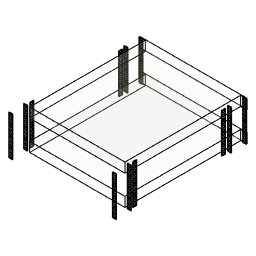
battery case (Autodesk Fusion 360 archive; units mm, degrees)
design "rack 19"
Autodesk Fusion 360 part; units mm, degrees
sketch "Sketch1" plane through (0, 0, 0) normal (0, 1, 0) x (1, 0, 0)
  line L0 (0, 0) -> (16.7, 0)
  line L1 (16.7, 0) -> (16.7, -177.8)
  line L2 (16.7, -177.8) -> (0, -177.8)
  line L3 (0, -177.8) -> (0, 0)
  line L4 (16.7, 0) -> (466.7, 0)
  line L5 (466.7, 0) -> (483.4, 0)
  line L6 (483.4, 0) -> (483.4, -177.8)
  line L7 (483.4, -177.8) -> (466.7, -177.8)
  line L8 (466.7, -177.8) -> (466.7, 0)
  line L9 (0, -88.9) -> (16.7, -88.9)
  line L10 (0, -88.9) -> (0, 0)
  line L11 (0, -44.45) -> (16.7, -44.45)
  line L12 (0, -88.9) -> (0, -177.8)
  line L13 (0, -133.35) -> (16.7, -133.35)
  line L14 (0, -88.9) -> (0, -44.45)
  line L15 (0, -66.675) -> (16.7, -66.675)
  line L16 (8.35, -66.675) -> (8.35, -82.55)
  line L17 (8.35, -66.675) -> (8.35, -50.8)
  line L18 (3.85, -87.05) -> (12.85, -87.05)
  line L19 (12.85, -87.05) -> (12.85, -78.05)
  line L20 (12.85, -78.05) -> (3.85, -78.05)
  line L21 (3.85, -78.05) -> (3.85, -87.05)
  line L22 (3.85, -87.05) -> (12.85, -78.05) construction
  line L23 (12.85, -87.05) -> (3.85, -78.05) construction
  line L24 (3.85, -71.175) -> (12.85, -71.175)
  line L25 (12.85, -71.175) -> (12.85, -62.175)
  line L26 (12.85, -62.175) -> (3.85, -62.175)
  line L27 (3.85, -62.175) -> (3.85, -71.175)
  line L28 (3.85, -71.175) -> (12.85, -62.175) construction
  line L29 (12.85, -71.175) -> (3.85, -62.175) construction
  line L30 (3.85, -55.3) -> (12.85, -55.3)
  line L31 (12.85, -55.3) -> (12.85, -46.3)
  line L32 (12.85, -46.3) -> (3.85, -46.3)
  line L33 (3.85, -46.3) -> (3.85, -55.3)
  line L34 (3.85, -55.3) -> (12.85, -46.3) construction
  line L35 (12.85, -55.3) -> (3.85, -46.3) construction
  line L36 (3.85, -10.85) -> (3.85, -1.85)
  line L37 (12.85, -42.6) -> (3.85, -42.6)
  line L38 (3.85, -17.725) -> (12.85, -26.725) construction
  line L39 (3.85, -33.6) -> (12.85, -33.6)
  line L40 (3.85, -1.85) -> (12.85, -10.85) construction
  line L41 (12.85, -1.85) -> (3.85, -10.85) construction
  line L42 (3.85, -33.6) -> (12.85, -42.6) construction
  line L43 (3.85, -1.85) -> (12.85, -1.85)
  line L44 (12.85, -10.85) -> (3.85, -10.85)
  line L45 (12.85, -17.725) -> (12.85, -26.725)
  line L46 (3.85, -17.725) -> (12.85, -17.725)
  line L47 (3.85, -26.725) -> (3.85, -17.725)
  line L48 (8.35, -22.225) -> (8.35, -38.1)
  line L49 (12.85, -17.725) -> (3.85, -26.725) construction
  line L50 (12.85, -33.6) -> (3.85, -42.6) construction
  line L51 (12.85, -1.85) -> (12.85, -10.85)
  line L52 (12.85, -33.6) -> (12.85, -42.6)
  line L53 (8.35, -22.225) -> (8.35, -6.35)
  line L54 (3.85, -42.6) -> (3.85, -33.6)
  line L55 (12.85, -26.725) -> (3.85, -26.725)
  line L56 (3.85, -166.95) -> (3.85, -175.95)
  line L57 (3.85, -90.75) -> (12.85, -99.75) construction
  line L58 (12.85, -99.75) -> (3.85, -99.75)
  line L59 (3.85, -131.5) -> (3.85, -122.5)
  line L60 (12.85, -166.95) -> (3.85, -166.95)
  line L61 (3.85, -90.75) -> (12.85, -90.75)
  line L62 (3.85, -99.75) -> (3.85, -90.75)
  line L63 (12.85, -106.625) -> (12.85, -115.625)
  line L64 (3.85, -160.075) -> (12.85, -160.075)
  line L65 (3.85, -135.2) -> (3.85, -144.2)
  line L66 (12.85, -175.95) -> (12.85, -166.95)
  line L67 (8.35, -111.125) -> (8.35, -127)
  line L68 (12.85, -122.5) -> (12.85, -131.5)
  line L69 (3.85, -106.625) -> (12.85, -106.625)
  line L70 (12.85, -106.625) -> (3.85, -115.625) construction
  line L71 (12.85, -160.075) -> (3.85, -151.075) construction
  line L72 (12.85, -90.75) -> (12.85, -99.75)
  line L73 (12.85, -90.75) -> (3.85, -99.75) construction
  line L74 (3.85, -175.95) -> (12.85, -166.95) construction
  line L75 (12.85, -175.95) -> (3.85, -166.95) construction
  line L76 (12.85, -122.5) -> (3.85, -131.5) construction
  line L77 (12.85, -115.625) -> (3.85, -115.625)
  line L78 (3.85, -144.2) -> (12.85, -144.2)
  line L79 (3.85, -122.5) -> (12.85, -131.5) construction
  line L80 (12.85, -135.2) -> (3.85, -135.2)
  line L81 (8.35, -155.575) -> (8.35, -139.7)
  line L82 (3.85, -122.5) -> (12.85, -122.5)
  line L83 (12.85, -131.5) -> (3.85, -131.5)
  line L84 (3.85, -115.625) -> (3.85, -106.625)
  line L85 (3.85, -175.95) -> (12.85, -175.95)
  line L86 (8.35, -155.575) -> (8.35, -171.45)
  line L87 (12.85, -160.075) -> (12.85, -151.075)
  line L88 (8.35, -111.125) -> (8.35, -95.25)
  line L89 (3.85, -160.075) -> (12.85, -151.075) construction
  line L90 (3.85, -144.2) -> (12.85, -135.2) construction
  line L91 (12.85, -144.2) -> (3.85, -135.2) construction
  line L92 (12.85, -151.075) -> (3.85, -151.075)
  line L93 (3.85, -106.625) -> (12.85, -115.625) construction
  line L94 (12.85, -144.2) -> (12.85, -135.2)
  line L95 (3.85, -151.075) -> (3.85, -160.075)
  line L96 (241.7, 0) -> (241.7, -10)
  line L97 (470.55, -122.5) -> (479.55, -131.5) construction
  line L98 (470.55, -78.05) -> (479.55, -78.05)
  line L99 (470.55, -106.625) -> (479.55, -115.625) construction
  line L100 (475.05, -111.125) -> (475.05, -127)
  line L101 (479.55, -122.5) -> (470.55, -131.5) construction
  line L102 (479.55, -122.5) -> (470.55, -122.5)
  line L103 (470.55, -106.625) -> (470.55, -115.625)
  line L104 (470.55, -166.95) -> (479.55, -166.95)
  line L105 (479.55, -87.05) -> (470.55, -87.05)
  line L106 (479.55, -115.625) -> (479.55, -106.625)
  line L107 (479.55, -87.05) -> (470.55, -78.05) construction
  line L108 (475.05, -22.225) -> (475.05, -6.35)
  line L109 (470.55, -62.175) -> (479.55, -62.175)
  line L110 (470.55, -115.625) -> (479.55, -115.625)
  line L111 (475.05, -111.125) -> (475.05, -95.25)
  line L112 (470.55, -55.3) -> (479.55, -46.3) construction
  line L113 (470.55, -71.175) -> (479.55, -62.175) construction
  line L114 (479.55, -10.85) -> (479.55, -1.85)
  line L115 (479.55, -166.95) -> (479.55, -175.95)
  line L116 (470.55, -55.3) -> (470.55, -46.3)
  line L117 (470.55, -175.95) -> (479.55, -166.95) construction
  line L118 (479.55, -1.85) -> (470.55, -1.85)
  line L119 (479.55, -26.725) -> (479.55, -17.725)
  line L120 (470.55, -42.6) -> (479.55, -42.6)
  line L121 (479.55, -55.3) -> (470.55, -46.3) construction
  line L122 (470.55, -175.95) -> (470.55, -166.95)
  line L123 (470.55, -131.5) -> (479.55, -131.5)
  line L124 (470.55, -144.2) -> (470.55, -135.2)
  line L125 (475.05, -66.675) -> (475.05, -50.8)
  line L126 (479.55, -62.175) -> (479.55, -71.175)
  line L127 (470.55, -160.075) -> (479.55, -151.075) construction
  line L128 (479.55, -71.175) -> (470.55, -71.175)
  line L129 (475.05, -155.575) -> (475.05, -139.7)
  line L130 (479.55, -151.075) -> (479.55, -160.075)
  line L131 (479.55, -175.95) -> (470.55, -175.95)
  line L132 (470.55, -135.2) -> (479.55, -135.2)
  line L133 (479.55, -1.85) -> (470.55, -10.85) construction
  line L134 (470.55, -17.725) -> (479.55, -26.725) construction
  line L135 (470.55, -90.75) -> (479.55, -99.75) construction
  line L136 (479.55, -135.2) -> (479.55, -144.2)
  line L137 (479.55, -106.625) -> (470.55, -106.625)
  line L138 (475.05, -22.225) -> (475.05, -38.1)
  line L139 (479.55, -90.75) -> (470.55, -90.75)
  line L140 (470.55, -10.85) -> (479.55, -10.85)
  line L141 (479.55, -42.6) -> (479.55, -33.6)
  line L142 (479.55, -33.6) -> (470.55, -42.6) construction
  line L143 (470.55, -1.85) -> (470.55, -10.85)
  line L144 (479.55, -160.075) -> (470.55, -160.075)
  line L145 (479.55, -90.75) -> (470.55, -99.75) construction
  line L146 (479.55, -99.75) -> (479.55, -90.75)
  line L147 (479.55, -55.3) -> (470.55, -55.3)
  line L148 (470.55, -122.5) -> (470.55, -131.5)
  line L149 (470.55, -26.725) -> (479.55, -26.725)
  line L150 (470.55, -160.075) -> (470.55, -151.075)
  line L151 (479.55, -144.2) -> (470.55, -144.2)
  line L152 (470.55, -71.175) -> (470.55, -62.175)
  line L153 (479.55, -78.05) -> (479.55, -87.05)
  line L154 (470.55, -87.05) -> (470.55, -78.05)
  line L155 (479.55, -46.3) -> (479.55, -55.3)
  line L156 (479.55, -144.2) -> (470.55, -135.2) construction
  line L157 (479.55, -131.5) -> (479.55, -122.5)
  line L158 (479.55, -71.175) -> (470.55, -62.175) construction
  line L159 (470.55, -151.075) -> (479.55, -151.075)
  line L160 (470.55, -144.2) -> (479.55, -135.2) construction
  line L161 (479.55, -160.075) -> (470.55, -151.075) construction
  line L162 (475.05, -155.575) -> (475.05, -171.45)
  line L163 (479.55, -175.95) -> (470.55, -166.95) construction
  line L164 (470.55, -17.725) -> (470.55, -26.725)
  line L165 (470.55, -87.05) -> (479.55, -78.05) construction
  line L166 (479.55, -106.625) -> (470.55, -115.625) construction
  line L167 (470.55, -99.75) -> (479.55, -99.75)
  line L168 (475.05, -66.675) -> (475.05, -82.55)
  line L169 (470.55, -90.75) -> (470.55, -99.75)
  line L170 (479.55, -33.6) -> (470.55, -33.6)
  line L171 (470.55, -1.85) -> (479.55, -10.85) construction
  line L172 (470.55, -33.6) -> (479.55, -42.6) construction
  line L173 (479.55, -17.725) -> (470.55, -26.725) construction
  line L174 (470.55, -33.6) -> (470.55, -42.6)
  line L175 (479.55, -17.725) -> (470.55, -17.725)
  line L176 (470.55, -46.3) -> (479.55, -46.3)
  point P0 (8.35, -82.55)
  point P1 (8.35, -66.675)
  point P2 (8.35, -50.8)
  point P3 (8.35, -22.225)
  point P4 (8.35, -6.35)
  point P5 (8.35, -38.1)
  point P6 (8.35, -171.45)
  point P7 (8.35, -95.25)
  point P8 (8.35, -111.125)
  point P9 (8.35, -139.7)
  point P10 (8.35, -155.575)
  point P11 (8.35, -127)
  point P12 (475.05, -95.25)
  point P13 (475.05, -111.125)
  point P14 (475.05, -155.575)
  point P15 (475.05, -66.675)
  point P16 (475.05, -127)
  point P17 (475.05, -6.35)
  point P18 (475.05, -82.55)
  point P19 (475.05, -22.225)
  point P20 (475.05, -50.8)
  point P21 (475.05, -139.7)
  point P22 (475.05, -38.1)
  point P23 (475.05, -171.45)
  dimension "d1" = 16.7
  dimension "d2" = 177.8
  dimension "d3" = 450
  dimension "d4" = 16.7
  dimension "d5" = 177.8
  dimension "d6" = 15.875
  dimension "d7" = 15.875
  dimension "d8" = 9
  dimension "d9" = 9
  dimension "d10" = 9
  dimension "d11" = 9
  dimension "d12" = 9
  dimension "d13" = 9
  constraint horizontal L0
  constraint vertical L1
  constraint horizontal L2
  constraint vertical L3
  constraint coincident L0.start L3.end
  constraint perpendicular L1 L4
  constraint horizontal L5
  constraint vertical L6
  constraint horizontal L7
  constraint vertical L8
  constraint midpoint L3 L9.start
  constraint midpoint L1 L9.end
  constraint midpoint L10 L11.start
  constraint coincident L1 L11.end
  constraint perpendicular L1 L11
  constraint midpoint L12 L13.start
  constraint coincident L1 L13.end
  constraint perpendicular L1 L13
  constraint midpoint L14 L15.start
  constraint coincident L1 L15.end
  constraint perpendicular L1 L15
  constraint midpoint L15 P1
  constraint perpendicular L15 L16
  constraint parallel L14 L17
  constraint horizontal L18
  constraint perpendicular L18 L19
  constraint parallel L18 L20
  constraint parallel L19 L21
  constraint coincident L22 P0
  constraint coincident L23 P0
  constraint coincident P0 L16.end
  constraint horizontal L24
  constraint perpendicular L24 L25
  constraint parallel L24 L26
  constraint parallel L25 L27
  constraint coincident L28 P1
  constraint coincident L29 P1
  constraint coincident P1 L16.start
  constraint horizontal L30
  constraint perpendicular L30 L31
  constraint parallel L30 L32
  constraint parallel L31 L33
  constraint coincident L34 P2
  constraint coincident L35 P2
  constraint coincident P2 L17.end
  constraint symmetric L11 P1 P3
  constraint symmetric L11 P0 P4
  constraint symmetric L11 P2 P5
  constraint symmetric L11 L18.start L36.end
  constraint symmetric L11 L18.end L41.start
  constraint symmetric L11 L19.end L40.end
  constraint symmetric L11 L20.end L36.start
  constraint symmetric L11 L24.start L38.start
  constraint symmetric L11 L24.end L45.start
  constraint symmetric L11 L25.end L38.end
  constraint symmetric L11 L26.end L47.start
  constraint symmetric L11 L30.start L39.start
  constraint symmetric L11 L30.end L39.end
  constraint symmetric L11 L31.end L37.start
  constraint symmetric L11 L32.end L37.end
  constraint symmetric L9 P1 P8
  constraint symmetric L9 P0 P7
  constraint symmetric L9 P2 P11
  constraint symmetric L9 L18.start L57.start
  constraint symmetric L9 L18.end L61.end
  constraint symmetric L9 L19.end L57.end
  constraint symmetric L9 L20.end L58.end
  constraint symmetric L9 L24.start L69.start
  constraint symmetric L9 L24.end L63.start
  constraint symmetric L9 L25.end L63.end
  constraint symmetric L9 L26.end L70.end
  constraint symmetric L9 L30.start L59.end
  constraint symmetric L9 L30.end L68.start
  constraint symmetric L9 L31.end L68.end
  constraint symmetric L9 L32.end L59.start
  constraint symmetric L9 L40.end L60.start
  constraint symmetric L9 L41.start L66.start
  constraint symmetric L9 L36.start L56.start
  constraint symmetric L9 L36.end L56.end
  constraint symmetric L9 P5 P9
  constraint symmetric L9 P3 P10
  constraint symmetric L9 L39.start L65.end
  constraint symmetric L9 P4 P6
  constraint symmetric L9 L45.start L64.end
  constraint symmetric L9 L38.start L64.start
  constraint symmetric L9 L38.end L87.end
  constraint symmetric L9 L47.start L71.end
  constraint symmetric L9 L37.end L65.start
  constraint symmetric L9 L37.start L80.start
  constraint symmetric L9 L39.end L78.end
  constraint midpoint L4 L96.start
  constraint perpendicular L4 L96
  constraint symmetric P1 L96 P15
  constraint symmetric P0 L96 P18
  constraint symmetric P2 L96 L125.end
  constraint symmetric L18.start L96 L105.start
  constraint symmetric L18.end L96 L105.end
  constraint symmetric L19.end L96 L98.start
  constraint symmetric L20.end L96 L98.end
  constraint symmetric L24.start L96 L126.end
  constraint symmetric L24.end L96 L113.start
  constraint symmetric L25.end L96 L109.start
  constraint symmetric L26.end L96 L109.end
  constraint symmetric L30.start L96 L121.start
  constraint symmetric L30.end L96 L112.start
  constraint symmetric L31.end L96 L116.end
  constraint symmetric L32.end L96 L112.end
  constraint symmetric P2 L96 P20
  constraint symmetric L40.end L96 L133.end
  constraint symmetric L41.start L96 L118.end
  constraint symmetric L36.start L96 L114.start
  constraint symmetric L36.end L96 L114.end
  constraint symmetric P5 L96 P22
  constraint symmetric P3 L96 P19
  constraint symmetric L39.start L96 L141.end
  constraint symmetric P4 L96 P17
  constraint symmetric L45.start L96 L134.start
  constraint symmetric L38.start L96 L119.end
  constraint symmetric L38.end L96 L149.start
  constraint symmetric L47.start L96 L119.start
  constraint symmetric L37.end L96 L120.end
  constraint symmetric L37.start L96 L120.start
  constraint symmetric L39.end L96 L170.end
  constraint symmetric L66.start L96 L117.start
  constraint symmetric L59.start L96 L97.end
  constraint symmetric L63.end L96 L103.end
  constraint symmetric L60.start L96 L104.start
  constraint symmetric L68.end L96 L101.end
  constraint symmetric L63.start L96 L99.start
  constraint symmetric P11 L96 P16
  constraint symmetric L56.end L96 L115.end
  constraint symmetric L65.end L96 L136.end
  constraint symmetric P10 L96 P14
  constraint symmetric L56.start L96 L104.end
  constraint symmetric L69.start L96 L106.end
  constraint symmetric P7 L96 P12
  constraint symmetric P9 L96 P21
  constraint symmetric P6 L96 P23
  constraint symmetric L64.start L96 L130.end
  constraint symmetric P8 L96 P13
  constraint symmetric L71.end L96 L127.end
  constraint symmetric L64.end L96 L127.start
  constraint symmetric L57.start L96 L139.start
  constraint symmetric L87.end L96 L150.end
  constraint symmetric L59.end L96 L101.start
  constraint symmetric L68.start L96 L97.start
  constraint symmetric L70.end L96 L99.end
  constraint symmetric L65.start L96 L132.end
  constraint symmetric L61.end L96 L135.start
  constraint symmetric L80.start L96 L124.end
  constraint symmetric L57.end L96 L145.end
  constraint symmetric L78.end L96 L124.start
  constraint symmetric L58.end L96 L135.end
  measures "d1" distance of L0.start L0.end
  measures "d2" distance of L0.start L2.end
  measures "d3" distance of L0.end L4.end
  measures "d4" distance of L4.end L5.end
  measures "d5" distance of L4.end L7.end
  measures "d6" distance of P1 P0
  measures "d7" distance of P1 P2
  measures "d8" distance of L19.end L20.end
  measures "d9" distance of L18.end L19.end
  measures "d10" distance of L25.end L26.end
  measures "d11" distance of L24.end L25.end
  measures "d12" distance of L31.end L32.end
  measures "d13" distance of L30.end L31.end
extrude "Extrude1" add sketch "Sketch1" against normal blind 2 contours L0 L1 L3 L10 L11 | L1 L3 L10 L11 L14 L15 L25 L26 L27 | L1 L3 L9 L10 L14 L15 L24 L25 L27 | L1 L3 L9 L12 L13 | L1 L2 L3 L12 L13 | L5 L6 L7 L8 makes body 1 at (9.85, 0, 59.8833) makes body 2 at (476.55, 0, 31.3083)
sketch "Sketch2" plane through (0, 0, 0) normal (0, 1, 0) x (1, 0, 0)
  line L0 (241.7, -0.5) -> (241.7, -10.5)
  line L1 (241.7, -0.5) -> (482.6, -0.5)
  line L2 (241.7, -0.5) -> (0.8, -0.5)
  line L3 (0.8, -0.5) -> (0.8, -44)
  line L4 (0.8, -44) -> (482.6, -44)
  line L5 (482.6, -44) -> (482.6, -0.5)
  line L6 (241.7, -44.95) -> (0.8, -44.95)
  line L7 (0.8, -44.95) -> (0.8, -88.45)
  line L8 (241.7, -44.95) -> (482.6, -44.95)
  line L9 (0.8, -88.45) -> (482.6, -88.45)
  line L10 (241.7, -44.95) -> (241.7, -54.95)
  line L11 (482.6, -88.45) -> (482.6, -44.95)
  line L12 (241.7, -133.85) -> (0.8, -133.85)
  line L13 (0.8, -133.85) -> (0.8, -177.35)
  line L14 (241.7, -133.85) -> (482.6, -133.85)
  line L15 (0.8, -177.35) -> (482.6, -177.35)
  line L16 (241.7, -133.85) -> (241.7, -143.85)
  line L17 (482.6, -177.35) -> (482.6, -133.85)
  line L18 (241.7, -0.5) -> (27.2, -0.5)
  line L19 (241.7, -0.5) -> (456.2, -0.5)
  line L20 (456.2, -0.5) -> (456.2, -44)
  line L21 (27.2, -0.5) -> (27.2, -44)
  line L22 (27.2, -44) -> (27.2, -177.35)
  line L23 (456.2, -44) -> (456.2, -177.35)
  point P0 (0, -44.45)
  point P1 (0, -133.35)
  dimension "d16" = 240.9
  dimension "d17" = 240.9
  dimension "d18" = 43.5
  dimension "d19" = 240.9
  dimension "d20" = 240.9
  dimension "d21" = 43.5
  dimension "d22" = 240.9
  dimension "d23" = 240.9
  dimension "d24" = 43.5
  dimension "d25" = 214.5
  dimension "d26" = 214.5
  constraint perpendicular L0 L1
  constraint perpendicular L0 L2
  constraint perpendicular L2 L3
  constraint perpendicular L3 L4
  constraint perpendicular L1 L5
  constraint perpendicular L8 L10
  constraint perpendicular L6 L10
  constraint perpendicular L6 L7
  constraint perpendicular L7 L9
  constraint perpendicular L8 L11
  constraint perpendicular L14 L16
  constraint perpendicular L12 L16
  constraint perpendicular L12 L13
  constraint perpendicular L13 L15
  constraint perpendicular L14 L17
  constraint perpendicular L0 L18
  constraint perpendicular L0 L19
  constraint coincident L4 L20.end
  constraint perpendicular L4 L20
  constraint coincident L4 L21.end
  constraint perpendicular L6 L21
  constraint coincident L15 L22.end
  constraint perpendicular L15 L22
  constraint coincident L15 L23.end
  constraint perpendicular L15 L23
  measures "d16" distance of L0.start L1.end
  measures "d17" distance of L0.start L2.end
  measures "d18" distance of L2.end L3.end
  measures "d19" distance of L6.start L8.end
  measures "d20" distance of L6.start L6.end
  measures "d21" distance of L7.end L6.end
  measures "d22" distance of L12.start L14.end
  measures "d23" distance of L12.start L12.end
  measures "d24" distance of L13.end L12.end
  measures "d25" distance of L0.start L18.end
  measures "d26" distance of L0.start L19.end
extrude "Extrude2" add sketch "Sketch2" along normal blind 2.5 separate body contours L1 L2 L4 L18 L19 L20 L21 | L1 L4 L5 L20 | L2 L3 L4 L21 | L6 L8 L9 L22 L23 | L8 L9 L11 L23 | L6 L7 L9 L22 | L12 L14 L15 L22 L23 | L14 L15 L17 L23 | L12 L13 L15 L22 makes body 3 at (161.4, 0, 15) makes body 4 at (161.4, 0, 59.45) makes body 5 at (161.4, 0, 148.35)
extrude "Extrude3" add sketch "Sketch2" against normal blind 230 contours L1 L2 L4 L18 L19 L20 L21 | L6 L8 L9 L22 L23 | L12 L14 L15 L22 L23 bodies 3 4 5
copy_body "CopyPasteBodies2" bodies 1 2 makes body 6 makes body 7
move_body "Move2" bodies 6 7 to x (1, 0, 0) y (0, 1, 0) z (0, 0, 1) at (0, -68, 0)
copy_body "CopyPasteBodies3" bodies 2 1 makes body 8 makes body 9
move_body "Move3" bodies 8 9 to x (1, 0, 0) y (0, 1, 0) z (0, 0, 1) at (0, -519, 0)
copy_body "CopyPasteBodies4" bodies 1 2 makes body 10 makes body 11
move_body "Move4" bodies 10 11 to x (1, 0, 0) y (0, 1, 0) z (0, 0, 1) at (0, -586, 0)
extrude "Extrude4" add 2 faces at (170.2, -230, 148.35) (170.2, -230, 29.5) along direction (0, -1, 0) blind 291 on bodies 3 5 bodies 5 3
sketch "Sketch3" plane through (0, 0, 0) normal (0, 0, 1) x (1, 0, 0)
  line L0 (466.7, -70) -> (466.7, -519)
  line L1 (466.7, -294.5) -> (466.7, -486)
  line L2 (466.7, -294.5) -> (466.7, -103)
  line L3 (16.7, -70) -> (16.7, -519)
  line L4 (466.7, -486) -> (16.7, -486)
  line L5 (466.7, -103) -> (16.7, -103)
  line L6 (12.85, -99.75) -> (3.85, -99.75)
  line L7 (8.35, -99.75) -> (16.15, -99.75)
  line L8 (16.15, -99.75) -> (11.15, -99.75)
  line L9 (11.15, -99.75) -> (11.15, -98.75)
  line L10 (16.7, -103) -> (11.15, -103)
  line L11 (16.7, -486) -> (11.15, -486)
  line L12 (466.7, -486) -> (472.25, -486)
  line L13 (466.7, -103) -> (472.25, -103)
  dimension "d33" = 191.5
  dimension "d34" = 191.5
  dimension "d35" = 7.8
  dimension "d36" = 5
  dimension "d37" = 1
  dimension "d38" = 5.55
  dimension "d39" = 5.55
  dimension "d40" = 5.55
  constraint vertical L0
  constraint midpoint L0 L1.start
  constraint parallel L0 L1
  constraint parallel L0 L2
  constraint parallel L0 L3
  constraint coincident L3 L4.end
  constraint perpendicular L3 L4
  constraint coincident L3 L5.end
  constraint perpendicular L3 L5
  constraint horizontal L6
  constraint midpoint L6 L7.start
  constraint parallel L6 L7
  constraint coincident L6 L8.end
  constraint perpendicular L7 L9
  constraint parallel L8 L10
  constraint perpendicular L3 L11
  constraint perpendicular L0 L12
  constraint perpendicular L0 L13
  measures "d33" distance of L1.start L1.end
  measures "d34" distance of L1.start L2.end
  measures "d35" distance of L7.start L7.end
  measures "d36" distance of L7.end L8.end
  measures "d37" distance of L8.end L9.end
  measures "d38" distance of L4.end L11.end
  measures "d39" distance of L1.end L12.end
  measures "d40" distance of L2.end L13.end
copy_body "CopyPasteBodies5" bodies 6 makes body 12
copy_body "CopyPasteBodies6" bodies 6 makes body 13
move_body "Move5" bodies 13 to x (0, 1, 0) y (-1, 0, 0) z (0, 0, 1) at (-58.85, -103, 0)
copy_body "CopyPasteBodies7" bodies 7 makes body 14
move_body "Move6" bodies 14 to x (0, 1, 0) y (-1, 0, 0) z (0, 0, 1) at (404.25, -569.7, 0)
copy_body "CopyPasteBodies8" bodies 13 14 makes body 15 makes body 16
move_body "Move7" bodies 15 16 to x (1, 0, 0) y (0, 1, 0) z (0, 0, 1) at (0, -399.7, 0)
hidden bodies 4
equation "d16 = ( 481.8 / 2 ) * 1 mm"
equation "d17 = ( 481.8 / 2 ) * 1 mm"
equation "d19 = ( 481.8 / 2 ) * 1 mm"
equation "d20 = ( 481.8 / 2 ) * 1 mm"
equation "d22 = ( 481.8 / 2 ) * 1 mm"
equation "d23 = ( 481.8 / 2 ) * 1 mm"
equation "d25 = ( 429 / 2 ) * 1 mm"
equation "d26 = ( 429 / 2 ) * 1 mm"
equation "d33 = ( 383 / 2 ) * 1 mm"
equation "d34 = ( 383 / 2 ) * 1 mm"

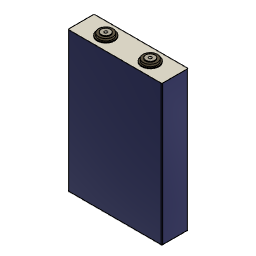
design "105Ah LiFePO4 cell"
Autodesk Fusion 360 part; units mm, degrees
sketch "Sketch1" plane through (0, 0, 0) normal (0, 0, 1) x (1, 0, 0)
  line L0 (0, 0) -> (131, 0)
  line L1 (131, 0) -> (131, 36.5)
  line L2 (131, 36.5) -> (0, 36.5)
  line L3 (0, 36.5) -> (0, 0)
  line L4 (65.5, 18.25) -> (96.5, 18.25)
  line L5 (65.5, 18.25) -> (34.5, 18.25)
  circle A0 centre (34.5, 18.25) radius 12
  circle A1 centre (96.5, 18.25) radius 12
  circle A2 centre (34.5, 18.25) radius 10
  circle A3 centre (96.5, 18.25) radius 10
  circle A4 centre (34.5, 18.25) radius 6.5
  circle A5 centre (96.5, 18.25) radius 6.5
  circle A6 centre (34.5, 18.25) radius 2
  circle A7 centre (96.5, 18.25) radius 2
  dimension "d1" = 131
  dimension "d2" = 36.5
  dimension "d3" = 31
  dimension "d4" = 31
  dimension "d5" = 24
  dimension "d6" = 24
  dimension "d7" = 20
  dimension "d8" = 20
  dimension "d9" = 13
  dimension "d10" = 13
  dimension "d17" = 4
  dimension "d18" = 4
  constraint horizontal L0
  constraint vertical L1
  constraint horizontal L2
  constraint vertical L3
  constraint coincident L0.start L3.end
  constraint perpendicular L3 L4
  constraint parallel L4 L5
  constraint coincident L5.end A0.centre
  constraint coincident L4.end A1.centre
  constraint concentric A0 A2
  constraint concentric A1 A3
  constraint concentric A0 A4
  constraint concentric A3 A5
  constraint concentric A2 A6
  constraint concentric A3 A7
  measures "d1" distance of L0.start L0.end
  measures "d2" distance of L0.start L2.end
  measures "d3" distance of L4.start L4.end
  measures "d4" distance of L4.start L5.end
  measures "d5" diameter of A0
  measures "d6" diameter of A1
  measures "d7" diameter of A2
  measures "d8" diameter of A3
  measures "d9" diameter of A4
  measures "d10" diameter of A5
  measures "d17" diameter of A6
  measures "d18" diameter of A7
extrude "Extrude1" add sketch "Sketch1" against normal blind 196 contours L0 L1 L2 L3 | A0 | A1 | A2 | A3 | A4 | A5 | A6 | A7
extrude "Extrude2" add sketch "Sketch1" along normal blind 1 contours A0 | A1
extrude "Extrude3" add sketch "Sketch1" along normal blind 4 contours A2 | A3
extrude "Extrude4" add sketch "Sketch1" along normal blind 5 contours A4 | A5
fillet "Fillet1" radius 1 4 edges at (0, 0, -98) (131, 0, -98) (131, 36.5, -98) (0, 36.5, -98) 1 faces at (43.6667, 12.1667, -196)
equation "d3 = ( 62 / 2 ) * 1 mm"
equation "d4 = ( 62 / 2 ) * 1 mm"
